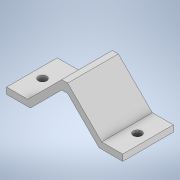
# Autodesk Inventor part: Fan_top
Saved by Autodesk Inventor 2022 (Build 260153000, 153)
## iProperties
Created: 2022-04-06
Part Number: Fan_top
Material: Generic
Document SubType Name: Modeling
Designer: Dani
Density: 1 g/cm^3
Appearance: Default
Author: Dani
## iProperties of the stored document Fan_top_3DPrint.ipt
Created: 2022-04-06
Part Number: Fan_top_3DPrint
Material: Generic
Document SubType Name: Modeling
Designer: Dani
Density: 1 g/cm^3
Appearance: Default
Author: Dani
Autodesk Inventor part; units mm, degrees
ref_plane "YZ Plane" through (0, 0, 0) normal (1, 0, 0) x (0, 1, 0)
ref_plane "XZ Plane" through (0, 0, 0) normal (0, 1, 0) x (-1, 0, 0)
ref_plane "XY Plane" through (0, 0, 0) normal (0, 0, 1) x (1, 0, 0)
sketch "Sketch1" plane through (0, 0, 0) normal (0, 0, 1) x (1, 0, 0)
  line L0 (0, -28.7085) -> (0, 28.7085) projected
  line L1 (0, 28.7085) -> (0, -28.7085) projected
  line L2 (-38.5085, 0) -> (38.5085, 0) projected
  line L3 (0, -16.2635) -> (16.2635, 0)
  line L4 (16.2635, 0) -> (0, 16.2635)
  line L5 (0, 16.2635) -> (-16.2635, 0)
  line L6 (-16.2635, 0) -> (0, -16.2635)
  line L7 (0, -16.2635) -> (0, 16.2635) construction
  line L8 (16.2635, 0) -> (-16.2635, 0) construction
  line L9 (0, -16.2635) -> (23, -16.2635) construction
  line L10 (0, -20.5061) -> (-17.5061, -3)
  line L11 (-17.5061, -3) -> (-27.5061, -3)
  line L12 (-27.5061, -3) -> (-27.5061, 3)
  line L13 (-27.5061, 3) -> (-17.5061, 3)
  line L14 (-17.5061, 3) -> (0, 20.5061)
  line L15 (0, 20.5061) -> (17.5061, 3)
  line L16 (17.5061, -3) -> (0, -20.5061)
  line L17 (-38.5085, 0) -> (38.5085, 0) projected
  line L18 (-27.5061, 0) -> (-16.2635, 0)
  line L19 (16.2635, 0) -> (23.5061, 0)
  line L20 (17.5061, -3) -> (27.5061, -3)
  line L21 (27.5061, -3) -> (27.5061, 3)
  line L22 (27.5061, 3) -> (17.5061, 3)
  line L23 (16.2635, 0) -> (27.5061, 0)
  point P0 (0, 0)
  point P1 (-16.2635, 0)
  point P2 (16.2635, 0)
  point P3 (27.5061, 0)
  dimension "d34" = 23
  dimension "d35" = 45
  dimension "d36" = 23
  dimension "d37" = 3
  dimension "d38" = 3
  dimension "d39" = 45
  dimension "d41" = 6
  dimension "d49" = 10
  dimension "d50" = 6
  dimension "d51" = 3
  dimension "d52" = 10
  constraints: 40 end point, 7 perpendicular, 6 midpoint, 3 horizontal, 3 parallel, 2 point on line, 1 equal length, 3 other
  measures "d34" distance of L3.start L3.end
  measures "d35" angle of L9 L3
  measures "d36" distance of L4.end L3.end
  measures "d37" distance between parallel lines of L10 L6
  measures "d38" distance between parallel lines of L14 L5
  measures "d39" angle of L0 L16
  measures "d41" distance between parallel lines of L13 L11
  measures "d49" distance from line of L12 L13.end
  measures "d50" distance between parallel lines of L20 L22
  measures "d51" distance between parallel lines of L20 L2
  measures "d52" distance of L21.end L15.end
extrude "Extrusion2" add sketch "Sketch1" along normal blind 24 contours L4 L0 L15 L22 L21 L2 | L2 L12 L13 L14 L0 L5
sketch "Sketch3" plane through (-27.5061, 3, 0) normal (0, 1, 0) x (1, 0, 0)
  line L0 (66.0146, 0) -> (-11.0024, 0) projected
  line L1 (0, 0) -> (0, -24) projected
  line L2 (55.0122, 0) -> (55.0122, -24) projected
  point P0 (27.5061, 0)
  point P1 (5, -12)
  point P2 (50.0122, -12)
  dimension "d55" = 12
  dimension "d56" = 12
  dimension "d57" = 5
  dimension "d58" = 5
  measures "d55" distance from line of L0 point (5, -12)
  measures "d56" distance from line of L0 point (50.012, -12)
  measures "d57" distance from line of L1 point (5, -12)
  measures "d58" distance from line of L2 point (50.012, -12)
hole "Hole1" at (-22.5061, 3, 12) at (22.5061, 3, 12) direction (0, -1, 0) diameter 4 end through all
chamfer "Chamfer1" distance 2 angle 45 2 edges at (0, 20.5061, 12) (0, 16.2635, 12)
body "Solid2"
